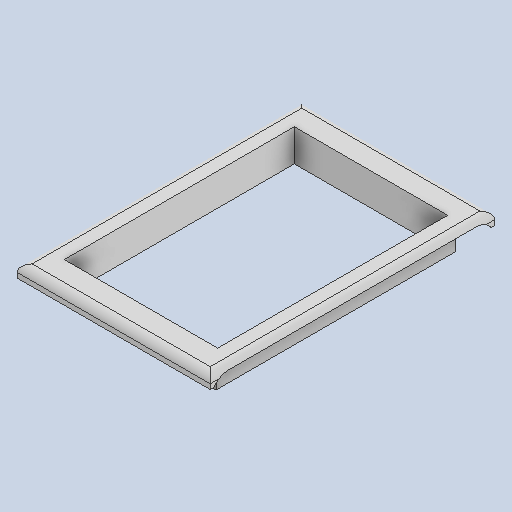
# Autodesk Inventor part: cage
Saved by Autodesk Inventor 2025 (Build 290162000, 162)
## iProperties
Created: 2025-07-16
Part Number: cage
Material: Generic
Document SubType Name: Modeling
Designer: Pravoslav
Density: 1 g/cm^3
Appearance: Default
Author: Pravoslav
Autodesk Inventor part; units mm, degrees
ref_plane "YZ Plane" through (0, 0, 0) normal (1, 0, 0) x (0, 1, 0)
ref_plane "XZ Plane" through (0, 0, 0) normal (0, 1, 0) x (-1, 0, 0)
ref_plane "XY Plane" through (0, 0, 0) normal (0, 0, 1) x (1, 0, 0)
sketch "Sketch1" plane through (0, 0, 0) normal (0, 1, 0) x (-1, 0, 0)
  line L0 (31, 46.5) -> (-31, 46.5)
  line L1 (-31, 46.5) -> (-31, -46.5)
  line L2 (-31, -46.5) -> (31, -46.5)
  line L3 (31, -46.5) -> (31, 46.5)
  line L4 (31, 46.5) -> (-31, -46.5) construction
  line L5 (-31, 46.5) -> (31, -46.5) construction
  line L6 (39, 57.5) -> (-39, 57.5)
  line L7 (-39, 57.5) -> (-39, -57.5)
  line L8 (-39, -57.5) -> (39, -57.5)
  line L9 (39, -57.5) -> (39, 57.5)
  line L10 (39, 57.5) -> (-39, -57.5) construction
  line L11 (-39, 57.5) -> (39, -57.5) construction
  point P0 (0, 0)
  dimension "d0" = 62
  dimension "d1" = 93
  dimension "d2" = 115
  dimension "d3" = 78
  constraints: 24 end point, 4 midpoint, 4 parallel, 2 horizontal, 2 perpendicular
  measures "d0" distance of L2.end L1.end
  measures "d1" distance of L1.end L0.end
  measures "d2" distance of L7.end L6.end
  measures "d3" distance between parallel lines of L7 L9
extrude "Extrusion1" add sketch "Sketch1" along normal blind 5
sketch "Sketch3" plane through (0, 0, 0) normal (0, -1, 0) x (1, 0, 0)
  line L0 (-39, -56) -> (39, -56)
  line L1 (39, -56) -> (39, 56)
  line L2 (39, 56) -> (-39, 56)
  line L3 (-39, 56) -> (-39, -56)
  line L4 (-39, -56) -> (39, 56) construction
  line L5 (39, -56) -> (-39, 56) construction
  point P0 (0, 0)
  dimension "d9" = 78
  dimension "d10" = 112
  constraints: 12 end point, 2 midpoint, 2 parallel, 1 horizontal, 1 perpendicular
  measures "d9" distance of L2.end L1.end
  measures "d10" distance of L1.end L0.end
extrude "Extrusion3" cut sketch "Sketch3" against normal blind 3
sketch "Sketch2" plane through (0, 0, 0) normal (0, -1, 0) x (1, 0, 0)
  line L0 (31, 46.5) -> (-31, 46.5) projected
  line L1 (-31, -46.5) -> (31, -46.5)
  line L2 (31, -46.5) -> (31, 46.5)
  line L3 (31, 46.5) -> (-31, 46.5)
  line L4 (-31, 46.5) -> (-31, -46.5)
  line L5 (-31, -46.5) -> (31, 46.5) construction
  line L6 (31, -46.5) -> (-31, 46.5) construction
  line L7 (-32.3333, -48.5) -> (32.3333, -48.5)
  line L8 (32.3333, -48.5) -> (32.3333, 48.5)
  line L9 (32.3333, 48.5) -> (-32.3333, 48.5)
  line L10 (-32.3333, 48.5) -> (-32.3333, -48.5)
  line L11 (-32.3333, -48.5) -> (32.3333, 48.5) construction
  line L12 (32.3333, -48.5) -> (-32.3333, 48.5) construction
  point P0 (0, 0)
  dimension "d17" = 2
  constraints: 24 end point, 4 midpoint, 4 parallel, 2 horizontal, 2 perpendicular, 1 point on line
  measures "d17" distance between parallel lines of L0 L9
extrude "Extrusion2" add sketch "Sketch2" along normal blind 8 and the other way blind 3
fillet "Fillet1" radius 6.75 2 edges at (0, 3, -56) (0, 3, 56)
fillet "Fillet2" radius 3 4 edges at (0, 5, -57.5) (39, 5, 0) (0, 5, 57.5) (-39, 5, 0)
body "Solid1"
